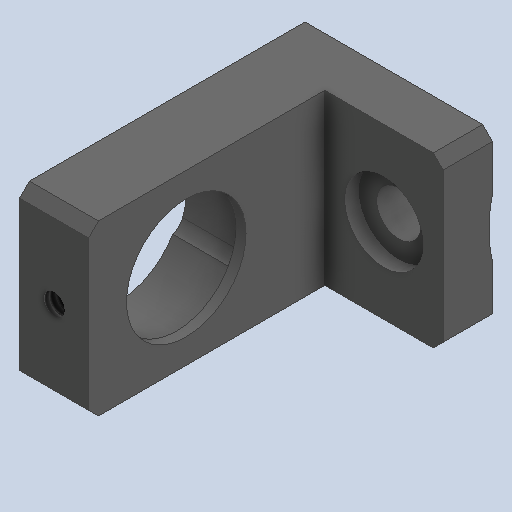
# Autodesk Inventor part: ADAPTER_fixed-mirror-BH19.05-D12.7
Saved by Autodesk Inventor 2024.2 (Build 282272000, 272)
## iProperties
ItemSpecifications: {"_id":"60468c71bf56440009da5009","finish":"543ef1f380da5b0c476373c1","finish_location":null,"material":"5515e170db035c20ce34af9a","process_initialism":null,"quotes":null,"current_quote":null,"quantity_ordered":1,"features":null,"hardware":null,"threading":{"quantity":1},"part_markings":[],"surface_roughness":null,"tolerance":null,"weld_quantity":null,"Notes":" :: Thread Spec: 1x See Notes/Drawing :: \r\n","certifications":[],"part":null,"revision_num":0,"last_history":null,"inspection_requirement_details":{"inspection_requirement":"std","customer_data_sheet":null},"feedback":null}
Created: 2021-02-12
Part Number: ADAPTER_fixed-mirror-BH19.05-D12.7
Material: Generic
Document SubType Name: Modeling
Designer: maria
Density: 1 g/cm^3
Appearance: Default(2)
Author: maria
Autodesk Inventor part; units mm, degrees
note: some values were not read from the file. Chosen so that the rebuilt part matches the saved one: direction of "Hole1"; direction of "Hole4".
ref_plane "YZ Plane" through (0, 0, 0) normal (1, 0, 0) x (0, 1, 0)
ref_plane "XZ Plane" through (0, 0, 0) normal (0, 1, 0) x (-1, 0, 0)
ref_plane "XY Plane" through (0, 0, 0) normal (0, 0, 1) x (1, 0, 0)
sketch "Sketch1" plane through (0, 0, 0) normal (0, 0, 1) x (1, 0, 0)
  line L0 (-7, 8.5625) -> (0, 8.5625)
  line L1 (0, 8.5625) -> (0, -8.5625)
  line L2 (0, -8.5625) -> (-7, -8.5625)
  line L3 (-7, -8.5625) -> (-7, 8.5625)
  point P0 (0, 0)
  dimension "d0" = 0
  dimension "FRONT_LENGTH" = 7
  dimension "WIDTH" = 17.125
  dimension "d3" = 8.5625
  constraints: 8 end point, 2 parallel, 1 horizontal, 1 perpendicular
  measures "d0" distance from line of point (0, 0) L1
  measures "FRONT_LENGTH" distance of L0.start L0.end
  measures "WIDTH" distance of L2.end L0.start
  measures "d3" distance from line of point (0, 0) L0
extrude "Extrusion1" add sketch "Sketch1" along normal blind 28.95
sketch "Sketch2" plane through (0, 0, 0) normal (0, 0, 1) x (1, 0, 0)
  line L0 (0, -8.5625) -> (0, 8.5625) projected
  line L1 (0, 8.5625) -> (12, 8.5625)
  line L2 (12, 8.5625) -> (12, -8.5625)
  line L3 (12, -8.5625) -> (0, -8.5625)
  line L4 (0, -8.5625) -> (0, 8.5625)
  point P0 (0, 0)
  point P1 (0, -8.5625)
  dimension "d6" = 17.125
  dimension "BACK_LENGTH" = 12
  constraints: 8 end point, 2 parallel, 1 horizontal, 1 perpendicular
  measures "d6" distance of L1.end L2.end
  measures "BACK_LENGTH" distance of L0.end L1.end
sketch "Sketch3" plane through (-7, -8.5625, 0) normal (-1, 0, 0) x (0, 0, 1)
  circle A0 centre (19.05, 8.5625) radius 6.5625
  circle A1 centre (19.05, 8.5625) radius 7.0705
  circle A2 centre (13.8389, 10.4592) radius 1.525
  circle A3 centre (13.8389, 6.6658) radius 1.525
  line L0 (13.8389, 10.4592) -> (19.05, 8.5625)
  line L1 (19.05, 8.5625) -> (13.8389, 6.6658)
  line L2 (19.05, 8.5625) -> (0, 8.5625)
  point P0 (12.4059, 6.1442)
  point P1 (13.4136, 5.2013)
  point P2 (13.4136, 11.9237)
  point P3 (12.4059, 10.9808)
  dimension "d8" = 0
  dimension "MIRROR_HOLE" = 13.125
  dimension "d10" = 14.141
  dimension "d11" = 3.05
  dimension "d12" = 3.05
  dimension "d13" = 19.05
  dimension "d14" = 20
  dimension "d15" = 20
  dimension "d16" = 0
  dimension "d17" = 0
  constraints: 6 end point, 4 centre point, 1 coincident
  measures "d8" vertical distance of L2.end A0.centre
  measures "MIRROR_HOLE" diameter of A0
  measures "d10" diameter of A1
  measures "d11" diameter of A2
  measures "d12" diameter of A3
  measures "d13" distance of L2.end A0.centre
  measures "d14" angle of L2 L1
  measures "d15" angle of L2 L0
extrude "Extrusion2" cut sketch "Sketch3" against normal blind 6 contours A0 A3 L1 L0 A2 | A2 A0 | A0 A2 | A3 A0 | A0 A3 | A2 L0 L2 A0 | A0 L2 A1 A2 | A3 A1 L2 A0 | A0 L2 L1 A3
sketch "Sketch5" plane through (-1, -8.5625, 0) normal (-1, 0, 0) x (0, 0, 1)
  circle A0 centre (19.05, 8.5625) radius 6.0625
  point P0 (0, 8.5625)
  dimension "d20" = 0
  dimension "d21" = 19.05
  dimension "d22" = 12.125
  constraints: 1 centre point
  measures "d20" vertical distance of point (0, 8.562) A0.centre
  measures "d21" distance of A0.centre point (0, 8.562)
  measures "d22" diameter of A0
extrude "Extrusion3" cut sketch "Sketch5" against normal up to surface (1 mm away)
extrude "Extrusion4" add sketch "Sketch2" along normal blind 5
sketch "Sketch6" plane through (0, 0, 5) normal (0, 0, 1) x (1, 0, 0)
  point P0 (0, 0)
  point P1 (6, 0)
  dimension "d27" = 0
  dimension "d28" = 6
  measures "d27" vertical distance of point (0, 0) point (6, 0)
  measures "d28" distance of point (0, 0) point (6, 0)
hole "Hole1" at (6, 0, 5) direction (0, 0, -1) diameter 4.5 depth 5 counterbore diameter 8 counterbore depth 1.5 clearance for "Socket Head Cap Screw" size "#8" standard "Ansi Unified Screw Threads"
sketch "Sketch7" plane through (0, 0, 0) normal (0, 0, -1) x (-1, 0, 0)
  circle A0 centre (-6, 0) radius 2.25 projected
  line L0 (-6, 5.498) -> (-6, 4.502) construction
  line L1 (-7.05, 5.498) -> (-7.05, 4.502)
  line L2 (-4.95, 4.502) -> (-4.95, 5.498)
  arc A1 (-4.95, 5.498) -> (-7.05, 5.498) centre (-6, 5.498) ccw
  arc A2 (-7.05, 4.502) -> (-4.95, 4.502) centre (-6, 4.502) ccw
  point P0 (0, 0)
  point P1 (-6, -5)
  point P2 (-6, 5)
  dimension "d36" = 0
  dimension "d37" = 0
  dimension "d38" = 5
  dimension "d39" = 5
  dimension "d63" = 1.05
  dimension "d64" = 0.996
  constraints: 8 end point, 4 point on circle, 4 tangent, 2 centre point, 1 midpoint, 1 parallel, 1 vertical
  measures "d36" horizontal distance of A0.centre point (-6, 5)
  measures "d37" horizontal distance of point (-6, -5) A0.centre
  measures "d38" distance of point (-6, -5) A0.centre
  measures "d39" distance of point (-6, 5) A0.centre
  measures "d63" radius of A2
  measures "d64" distance of L0.start L0.end
hole "Hole2" at (6, -5, 0) direction (0, 0, 1) diameter 2.1 depth 2.1
sketch "Sketch8" plane through (0, 0, 28.95) normal (0, 0, 1) x (1, 0, 0)
  point P0 (0, 0)
  point P1 (-3.5, 0)
  dimension "d47" = 3.5
  dimension "d48" = 0
  measures "d47" distance of point (0, 0) point (-3.5, 0)
  measures "d48" vertical distance of point (0, 0) point (-3.5, 0)
hole "Hole4" at (-3.5, 0, 28.95) direction (0, 0, -1) diameter 2.1565 end up to surface thread size "4-40 UNC" class "3B" standard "ANSI Unified Screw Threads"
extrude "Extrusion5" cut sketch "Sketch7" against normal blind 2.1 contours A1 L2 A2 L1
chamfer "Chamfer1" distance 1 angle 45 4 edges at (-3.5, -8.5625, 28.95) (-3.5, 8.5625, 28.95) (12, -8.5625, 2.5) (12, 8.5625, 2.5)
sketch "Sketch9" plane through (12, -7.5625, 0) normal (1, 0, 0) x (0, 0, -1)
  circle A0 centre (12.35, 7.5625) radius 12.7
  point P0 (0, 7.5625)
  dimension "d70" = 0
  dimension "d71" = 25.4
  dimension "d72" = 12.35
  constraints: 1 centre point
  measures "d70" vertical distance of A0.centre point (0, 7.562)
  measures "d71" diameter of A0
  measures "d72" distance of A0.centre point (0, 7.562)
extrude "Extrusion6" cut sketch "Sketch9" against normal up to surface (19 mm away)
equation "\"WIDTH\" = MIRROR_HOLE + 2 * MIN_WALL_THICKNESS"
equation "\"d3\" = 0.5 * WIDTH"
equation "\"d13\" = BEAM_HEIGHT"
equation "\"d6\" = WIDTH"
equation "\"d21\" = BEAM_HEIGHT"
equation "\"d28\" = 0.5 * BACK_LENGTH"
equation "\"d39\" = d38"
equation "\"d47\" = 0.5 * FRONT_LENGTH"
equation "\"BEAM_HEIGHT\" = 19.05"
equation "\"MIN_WALL_THICKNESS\" = 2"
equation "\"OPTICS_DIAMETER\" = 12.7"
equation "\"TOLERANCE\" = 0.05"
body "Solid1"
